Drive Bearing Hub_v1 (Autodesk Fusion 360 design; units mm, degrees)
Autodesk Fusion 360 part; units mm, degrees
sketch "Sketch1" plane through (0, 0, 0) normal (0, 0, 1) x (1, 0, 0)
  circle A0 centre (0, 0) radius 11.2
  circle A1 centre (0, 0) radius 5.15
  circle A2 centre (0, 0) radius 1.5
  dimension "d1" = 22.4
  dimension "d2" = 10.3
  dimension "d3" = 3
  constraint coincident A0.centre A1.centre
  constraint concentric A0 A1
  measures "d1" diameter of A0
  measures "d2" diameter of A1
  measures "d3" diameter of A2
extrude "Extrude1" add sketch "Sketch1" along normal blind 1 contours A0 | A1 makes body 1
extrude "Extrude2" add sketch "Sketch1" along normal blind 4 separate body contours A1 makes body 2
sketch "Sketch2" plane through (0, 0, 4) normal (0, 0, 1) x (-1, 0, 0)
  circle A0 centre (0, 0) radius 1.5
  circle A1 centre (0, 0) radius 5.15
  circle A2 centre (0, 0) radius 2.5
  dimension "d8" = 5
  constraint coincident A0.centre A1.centre
  measures "d8" diameter of A2
extrude "Extrude3" cut sketch "Sketch2" against normal blind 3 contours A2 bodies 2
